Autodesk Inventor part; units mm, degrees
(part 2 of 2)
sketch "Sketch2" plane through (-209.3721, -28.8511, 0) normal (0, 0, -1) x (-1, 0, 0)
  line L0 (-33.637, 21.3645) -> (-33.637, 17.6082) projected
  line L1 (-48.637, 21.3645) -> (-33.637, 21.3645) projected
  line L2 (-48.637, 17.6082) -> (-48.637, 21.3645) projected
  line L3 (-48.637, 17.6082) -> (-33.637, 17.6082) projected
  line L4 (-49.637, 20.8382) -> (-49.637, 18.1345) projected
  line L5 (-32.637, 18.1345) -> (-32.637, 20.8382) projected
  line L6 (-26.637, 21.1086) -> (-26.637, 17.8642) projected
  line L7 (-25.437, 17.2326) -> (-25.437, 21.7402) projected
  line L8 (-4.837, 21.7402) -> (-4.837, 17.2326) projected
  line L9 (-25.437, 21.7402) -> (-4.837, 21.7402) projected
  line L10 (-25.437, 17.2326) -> (-25.437, 21.7402) projected
  line L11 (-25.437, 17.2326) -> (-4.837, 17.2326) projected
  line L12 (-3.637, 17.8642) -> (-3.637, 21.1086) projected
  line L13 (2.363, 17.6864) -> (2.363, 21.2864) projected
  spline S0 degree 2 poles (3.563, 17.2326) (3.5291, 17.2777) (2.2161, 19.0571) (2.9463, 20.9193) (3.563, 21.7402) knots 3.326026 3.326026 3.326026 3.405258 7.652604 9.28848 9.28848 9.28848 weights 9.554217 9.619621 13.096193 10.904595 9.554217 projected
  line L14 (3.563, 17.2326) -> (46.163, 17.2326) projected
  line L15 (46.163, 21.7402) -> (46.163, 17.2326) projected
  line L16 (3.563, 21.7402) -> (46.163, 21.7402) projected
  line L17 (47.363, 21.2864) -> (47.363, 17.6864) projected
  circle A0 centre (29.9929, 5.3328) radius 3.7 projected
  circle A1 centre (29.9929, 5.3328) radius 5.3 projected
  circle A2 centre (29.9929, 5.3328) radius 5.8 projected
  circle A3 centre (45.4783, 5.604) radius 5.8 projected
  circle A4 centre (45.4783, 5.604) radius 5.3 projected
  line L18 (2.363, 14.1086) -> (2.363, 10.8642) projected
  line L19 (18.363, 10.8642) -> (18.363, 14.1086) projected
  line L20 (18.363, 3.8642) -> (18.363, 7.1086) projected
  line L21 (2.363, 7.1086) -> (2.363, 3.8642) projected
  line L22 (-3.637, 10.8642) -> (-3.637, 14.1086) projected
  line L23 (-26.637, 14.1086) -> (-26.637, 10.8642) projected
  line L24 (-26.637, 7.1086) -> (-26.637, 3.8642) projected
  line L25 (-3.637, 3.8642) -> (-3.637, 7.1086) projected
  line L26 (-3.637, -3.1358) -> (-3.637, 0.1086) projected
  line L27 (-26.637, 0.1086) -> (-26.637, -3.1358) projected
  line L28 (-32.637, 0.1345) -> (-32.637, 2.8382) projected
  line L29 (-32.637, 6.1345) -> (-32.637, 8.8382) projected
  line L30 (-32.637, 12.1345) -> (-32.637, 14.8382) projected
  line L31 (-49.637, 14.8382) -> (-49.637, 12.1345) projected
  line L32 (-49.637, 8.8382) -> (-49.637, 6.1345) projected
  line L33 (-49.637, 2.8382) -> (-49.637, 0.1345) projected
  circle A5 centre (-40.7352, -15) radius 3.15 projected
  circle A6 centre (-26.7352, -15) radius 3.15 projected
  arc A7 (-40.7352, -11.1) -> (-40.7352, -18.9) centre (-40.7352, -15) ccw projected
  line L34 (-40.7352, -18.9) -> (-26.7352, -18.9) projected
  arc A8 (-26.7352, -18.9) -> (-26.7352, -11.1) centre (-26.7352, -15) ccw projected
  line L35 (-26.7352, -11.1) -> (-40.7352, -11.1) projected
  arc A9 (-40.7352, -10.5) -> (-40.7352, -19.5) centre (-40.7352, -15) ccw projected
  arc A10 (-26.7352, -19.5) -> (-26.7352, -10.5) centre (-26.7352, -15) ccw projected
  arc A11 (-3.0622, -10.5) -> (-3.0622, -19.5) centre (-3.0622, -15) ccw projected
  circle A12 centre (-3.0622, -15) radius 3.15 projected
  circle A13 centre (10.9378, -15) radius 3.15 projected
  arc A14 (-3.0622, -11.1) -> (-3.0622, -18.9) centre (-3.0622, -15) ccw projected
  line L36 (10.9378, -18.9) -> (-3.0622, -18.9) projected
  arc A15 (10.9378, -18.9) -> (10.9378, -11.1) centre (10.9378, -15) ccw projected
  line L37 (-3.0622, -11.1) -> (10.9378, -11.1) projected
  arc A16 (10.9378, -19.5) -> (10.9378, -10.5) centre (10.9378, -15) ccw projected
  line L38 (25.5408, -13.2) -> (26.1532, -13.8124) projected
  line L39 (25.5408, -13.2) -> (22.9656, -13.2) projected
  line L40 (22.3532, -13.8124) -> (22.9656, -13.2) projected
  line L41 (22.3532, -13.8124) -> (22.3532, -16.3876) projected
  line L42 (22.9656, -17) -> (22.3532, -16.3876) projected
  line L43 (22.9656, -17) -> (25.5408, -17) projected
  line L44 (26.1532, -16.3876) -> (25.5408, -17) projected
  line L45 (26.1532, -16.3876) -> (26.1532, -13.8124) projected
  line L46 (33.3532, -16.3876) -> (32.7408, -17) projected
  line L47 (33.3532, -16.3876) -> (33.3532, -13.8124) projected
  line L48 (32.7408, -13.2) -> (33.3532, -13.8124) projected
  line L49 (32.7408, -13.2) -> (30.1656, -13.2) projected
  line L50 (29.5532, -13.8124) -> (30.1656, -13.2) projected
  line L51 (29.5532, -13.8124) -> (29.5532, -16.3876) projected
  line L52 (30.1656, -17) -> (29.5532, -16.3876) projected
  line L53 (30.1656, -17) -> (32.7408, -17) projected
  line L54 (-50, -27.5) -> (50, -27.5) projected
  arc A17 (50, -27.5) -> (60, -17.5) centre (50, -17.5) ccw projected
  line L55 (60, -17.5) -> (60, 17.5) projected
  arc A18 (60, 17.5) -> (50, 27.5) centre (50, 17.5) ccw projected
  line L56 (50, 27.5) -> (-50, 27.5) projected
  arc A19 (-50, 27.5) -> (-60, 17.5) centre (-50, 17.5) ccw projected
  line L57 (-60, 17.5) -> (-60, -17.5) projected
  arc A20 (-60, -17.5) -> (-50, -27.5) centre (-50, -17.5) ccw projected
  line L58 (-60, 19.9645) -> (-60, 18.9645)
  line L59 (60, 18.9645) -> (60, 19.9645)
  line L60 (-60, 5.0086) -> (-60, 6.0086)
  line L61 (60, 6.0086) -> (60, 5.0086)
  line L62 (51.2642, 6.0086) -> (60, 6.0086)
  line L63 (60, 5.0086) -> (51.2477, 5.0086)
  line L64 (35.7534, 6.0086) -> (39.6925, 6.0086)
  line L65 (39.709, 5.0086) -> (35.7838, 5.0086)
  line L66 (24.2019, 5.0086) -> (18.363, 5.0086)
  line L67 (18.363, 6.0086) -> (24.2324, 6.0086)
  line L68 (-30.137, 19.9645) -> (-29.137, 19.9645)
  line L69 (-29.137, 19.9645) -> (-29.137, -2.0358)
  line L70 (-29.137, -2.0358) -> (-30.137, -2.0358)
  line L71 (-30.137, -2.0358) -> (-30.137, 19.9645)
  line L72 (18.363, 12.0086) -> (60, 12.0086)
  line L73 (60, 12.0086) -> (60, 13.0086)
  line L74 (60, 13.0086) -> (18.363, 13.0086)
  line L75 (18.363, 13.0086) -> (18.363, 12.0086)
  line L76 (-29.137, 12.0086) -> (-29.137, 13.0086)
  line L77 (18.363, 13.0086) -> (18.363, 12.0086)
  line L78 (-3.637, 4.9642) -> (2.5322, 4.9642)
  line L79 (2.5322, 4.9642) -> (2.5322, 5.9642)
  line L80 (2.5322, 5.9642) -> (-3.637, 5.9642)
  line L81 (-3.637, 5.9642) -> (-3.637, 4.9642)
  line L82 (-26.637, 4.9642) -> (-30.137, 4.9642)
  line L83 (-30.137, 4.9642) -> (-30.137, 5.9642)
  line L84 (-30.137, 5.9642) -> (-26.637, 5.9642)
  line L85 (-26.637, 5.9642) -> (-26.637, 4.9642)
  line L86 (-26.637, -1.0358) -> (-29.137, -1.0358)
  line L87 (-29.137, -1.0358) -> (-29.137, -2.0358)
  line L88 (-29.137, -2.0358) -> (-26.637, -2.0358)
  line L89 (-26.637, -2.0358) -> (-26.637, -1.0358)
  line L90 (-32.637, 1.9882) -> (-29.137, 1.9882)
  line L91 (-29.137, 1.9882) -> (-29.137, 0.9882)
  line L92 (-29.137, 0.9882) -> (-32.637, 0.9882)
  line L93 (-32.637, 0.9882) -> (-32.637, 1.9882)
  line L94 (-32.637, 7.9882) -> (-29.137, 7.9882)
  line L95 (-29.137, 7.9882) -> (-29.137, 6.9882)
  line L96 (-29.137, 6.9882) -> (-32.637, 6.9882)
  line L97 (-32.637, 6.9882) -> (-32.637, 7.9882)
  line L98 (-32.637, 13.9882) -> (-30.137, 13.9882)
  line L99 (-30.137, 13.9882) -> (-30.137, 12.9882)
  line L100 (-30.137, 12.9882) -> (-32.637, 12.9882)
  line L101 (-32.637, 12.9882) -> (-32.637, 13.9882)
  line L102 (-49.637, 13.9882) -> (-60, 13.9882)
  line L103 (-60, 13.9882) -> (-60, 12.9882)
  line L104 (-60, 12.9882) -> (-49.637, 12.9882)
  line L105 (-32.637, 12.9882) -> (-32.637, 13.9882)
  line L106 (-49.637, 7.9882) -> (-60, 7.9882)
  line L107 (-60, 7.9882) -> (-60, 6.9882)
  line L108 (-60, 6.9882) -> (-49.637, 6.9882)
  line L109 (-32.637, 6.9882) -> (-32.637, 7.9882)
  line L110 (-49.637, 1.9882) -> (-60, 1.9882)
  line L111 (-60, 1.9882) -> (-60, 0.9882)
  line L112 (-60, 0.9882) -> (-49.637, 0.9882)
  line L113 (-0.437, 27.5) -> (-1.637, 27.5)
  line L114 (-1.637, 27.5) -> (-1.637, -2.0358)
  line L115 (-1.637, -2.0358) -> (-0.437, -2.0358)
  line L116 (-0.437, -2.0358) -> (-0.437, 27.5)
  line L117 (-3.637, -1.0358) -> (-1.637, -1.0358)
  line L118 (-1.637, -1.0358) -> (-1.637, -2.0358)
  line L119 (-1.637, -2.0358) -> (-3.637, -2.0358)
  line L120 (-3.637, -2.0358) -> (-3.637, -1.0358)
  line L121 (47.363, 18.9645) -> (60, 18.9645)
  line L122 (60, 19.9645) -> (47.363, 19.9645)
  line L123 (-29.137, 13.0086) -> (-26.637, 13.0086)
  line L124 (-3.637, 13.0086) -> (2.363, 13.0086)
  line L125 (2.363, 12.0086) -> (-3.637, 12.0086)
  line L126 (-26.637, 12.0086) -> (-29.137, 12.0086)
  line L127 (2.363, 19.9645) -> (-4.837, 19.9645)
  line L128 (-4.837, 18.9645) -> (2.363, 18.9645)
  line L129 (-25.437, 19.9645) -> (-32.637, 19.9645)
  line L130 (-49.637, 19.9645) -> (-60, 19.9645)
  line L131 (-60, 18.9645) -> (-49.637, 18.9645)
  line L132 (-32.637, 18.9645) -> (-25.437, 18.9645)
  line L133 (60, -15.5) -> (60, -14.5)
  line L134 (-60, -14.5) -> (-60, -15.5)
  line L135 (-14.2622, -14.5) -> (-13.0622, -14.5)
  line L136 (-13.0622, -14.5) -> (-13.0622, -27.5)
  line L137 (-13.0622, -27.5) -> (-14.2622, -27.5)
  line L138 (-14.2622, -27.5) -> (-14.2622, -14.5)
  line L139 (18.1532, -14.5) -> (19.3532, -14.5)
  line L140 (19.3532, -14.5) -> (19.3532, -27.5)
  line L141 (19.3532, -27.5) -> (18.1532, -27.5)
  line L142 (18.1532, -27.5) -> (18.1532, -14.5)
  line L143 (50.8547, -15.5) -> (60, -15.5)
  line L144 (39.8194, -14.5) -> (33.3532, -14.5)
  line L145 (33.3532, -15.5) -> (39.8336, -15.5)
  line L146 (29.5532, -14.5) -> (26.1532, -14.5)
  line L147 (26.1532, -15.5) -> (29.5532, -15.5)
  line L148 (22.3532, -14.5) -> (15.41, -14.5)
  line L149 (15.41, -15.5) -> (22.3532, -15.5)
  line L150 (-60, -15.5) -> (-45.2073, -15.5)
  line L151 (-7.5343, -14.5) -> (-22.2631, -14.5)
  line L152 (-45.2073, -14.5) -> (-60, -14.5)
  line L153 (-22.2631, -15.5) -> (-7.5343, -15.5)
  circle A21 centre (45.2028, -14.9239) radius 5.4 projected
  line L154 (60, -15.5) -> (50.5719, -15.5)
  line L155 (50.5861, -14.5) -> (60, -14.5)
  line L156 (60, -14.5) -> (60, -15.5)
  point P0 (-209.3721, 28.8511)
  point P1 (-30.887, 6.9882)
  point P2 (-14.2622, -21)
  point P3 (18.1532, -15.5)
  point P4 (18.1532, -27.5)
  point P5 (19.3532, -15.5)
  point P6 (19.3532, -14.5)
  point P7 (-14.2622, -15.5)
  point P8 (-14.2622, -27.5)
  point P9 (-13.0622, -15.5)
  point P10 (-13.0622, -14.5)
  point P11 (-60, -14.5)
  point P12 (-60, -15.5)
  point P13 (-60, 1.9882)
  point P14 (-60, 7.9882)
  point P15 (-60, 13.9882)
  point P16 (-59.8922, 18.9645)
  point P17 (-59.6915, 19.9645)
  point P18 (-29.137, -2.0358)
  point P19 (-26.637, -2.0358)
  point P20 (-29.137, -1.0358)
  point P21 (-29.137, 4.9642)
  point P22 (-26.637, 5.9642)
  point P23 (-29.137, 5.9642)
  point P24 (-29.137, 12.0086)
  point P25 (-29.137, 18.9645)
  point P26 (-26.637, 18.9645)
  point P27 (-26.637, 19.9645)
  point P28 (-29.137, 19.9645)
  point P29 (-30.137, 18.9645)
  point P30 (-30.137, 13.9882)
  point P31 (-32.637, 12.9882)
  point P32 (-30.137, 7.9882)
  point P33 (-32.637, 6.9882)
  point P34 (-30.137, 6.9882)
  point P35 (-30.137, 1.9882)
  point P36 (-32.637, 0.9882)
  point P37 (-30.137, 0.9882)
  point P38 (-0.437, 5.9642)
  point P39 (-0.437, 12.0086)
  point P40 (-0.437, 13.0086)
  point P41 (-0.437, 18.9645)
  point P42 (-0.437, 19.9645)
  point P43 (-1.637, 27.5)
  point P44 (-1.637, 19.9645)
  point P45 (-3.637, 19.9645)
  point P46 (-3.637, 18.9645)
  point P47 (-1.637, 18.9645)
  point P48 (-1.637, 13.0086)
  point P49 (-1.637, 12.0086)
  point P50 (-1.637, 5.9642)
  point P51 (-3.637, 5.9642)
  point P52 (-1.637, 4.9642)
  point P53 (-1.637, -1.0358)
  point P54 (-3.637, -2.0358)
  point P55 (-1.637, -2.0358)
  point P56 (-0.437, 4.9642)
  point P57 (59.6915, 19.9645)
  point P58 (59.8922, 18.9645)
  point P59 (18.363, 13.0086)
  point P60 (60, 12.0086)
  point P61 (60, 5.0086)
  point P62 (60, 6.0086)
  point P63 (60, -14.5)
  point P64 (50.8547, -15.5)
  point P65 (60, -15.5)
  point P66 (2.363, 4.9642)
  point P67 (2.363, 5.9642)
  dimension "d79" = 1
  dimension "d80" = 2.5
  dimension "d81" = 2.5
  dimension "d82" = 1
  dimension "d83" = 1.1
  dimension "d84" = 1.1444
  dimension "d85" = 1
  dimension "d86" = 1.1
  dimension "d87" = 1
  dimension "d89" = 1.2
  dimension "d90" = 2
  dimension "d91" = 1
  dimension "d92" = 0.85
  dimension "d93" = 0.8537
  dimension "d94" = 1
  dimension "d95" = 0.85
  dimension "d96" = 1
  dimension "d97" = 0.85
  dimension "d98" = 1
  dimension "d99" = 1.1
  dimension "d100" = 1.1444
  dimension "d101" = 1.1
  dimension "d102" = 1
  dimension "d103" = 1.1
  dimension "d104" = 1.1444
  dimension "d105" = 1.1444
  dimension "d106" = 1
  dimension "d107" = 0.8737
  dimension "d111" = 1.2
  dimension "d112" = 1.2
  dimension "d113" = 3
  dimension "d114" = 10
  dimension "d115" = 1
  dimension "d116" = 3.4
  dimension "d117" = 3.4
  dimension "d118" = 1
  constraints: 198 end point, 93 parallel, 62 point on line, 31 horizontal, 30 perpendicular, 27 horizontal alignment, 20 point on circle, 6 vertical alignment, 3 coincident, 2 midpoint
  measures "d79" distance between parallel lines of L69 L71
  measures "d80" distance between parallel lines of L5 L71
  measures "d81" distance between parallel lines of L69 L6
  measures "d82" distance between parallel lines of L72 L74
  measures "d83" distance from line of L19.end L74
  measures "d84" distance from line of L72 L19.start
  measures "d85" distance between parallel lines of L119 L117
  measures "d86" distance from line of L119 L26.start
  measures "d87" distance between parallel lines of L78 L80
  measures "d89" distance between parallel lines of L116 L114
  measures "d90" distance between parallel lines of L12 L114
  measures "d91" distance between parallel lines of L100 L98
  measures "d92" distance from line of L30.end L98
  measures "d93" distance from line of L100 L30.start
  measures "d94" distance from line of point (-30.887, 6.988) L94
  measures "d95" distance from line of L29.end L94
  measures "d96" distance between parallel lines of L92 L90
  measures "d97" distance of L28.end L90.start
  measures "d98" distance between parallel lines of L86 L88
  measures "d99" distance from line of L27.end L88
  measures "d100" distance of L27.start L86.start
  measures "d101" distance from line of L82 L24.end
  measures "d102" distance between parallel lines of L66 L67
  measures "d103" distance of L20.end L67.start
  measures "d104" distance from line of L20.start L66
  measures "d105" distance from line of L21.start L80
  measures "d106" distance between parallel lines of L131 L130
  measures "d107" distance from line of L4.start L130
  measures "d111" distance from line of L136 point (-14.262, -21)
  measures "d112" distance between parallel lines of L140 L142
  measures "d113" distance between parallel lines of L41 L140
  measures "d114" distance from line of A14.centre L136
  measures "d115" distance between parallel lines of L150 L152
  measures "d116" distance between parallel lines of L35 L152
  measures "d117" distance between parallel lines of L34 L150
  measures "d118" distance between parallel lines of L155 L143
extrude "Extrusion2" add sketch "Sketch2" against normal blind 1 contours L4 L131 A19 L130 | L56 L116 L127 L114 | L102 L31 L104 L57 | L127 L116 L128 L114 | L114 L128 L12 L127 | L127 L13 L128 L116 | L128 L116 L124 L114 | L106 L32 L108 L57 | A18 L121 L17 L122 | L124 L116 L125 L114 | L114 L125 L22 L124 | L124 L18 L125 L116 | L125 L116 L80 L114 | L114 L78 L25 L80 | L80 L116 L78 L114 | L55 L72 L19 L74 | L80 L21 L78 L116 | L78 L116 L115 L114 | L110 L33 L112 L57 | L114 L119 L26 L117 | L6 L132 L69 L129 | L55 L63 A3 L62 | L69 L132 L71 L68 | L152 A9 L150 L57 | L69 L94 L71 L132 | L71 L132 L5 L129 | L55 L143 L154 A21 L155 | A3 L65 A2 L64 | L123 L23 L126 L69 | L71 L100 L30 L98 | A21 L145 L47 L144 | A2 L66 L20 L67 | L69 L96 L71 L94 | L138 L153 L136 L54 | L69 L84 L71 L96 | L71 L96 L29 L94 | L153 A10 L151 L138 | L138 L135 L136 L153 | L54 L142 L149 L140 | L84 L24 L82 L69 | L69 L82 L71 L84 | L136 L151 A11 L153 | L149 L142 L139 L140 | L140 L148 L41 L149 | L69 L90 L71 L82 | L149 A16 L148 L142 | L69 L92 L71 L90 | L69 L70 L71 L92 | L71 L92 L28 L90 | L51 L147 L45 L146 | L86 L27 L88 L69
sketch "Sketch3" plane through (-357.3721, -11.3511, 0) normal (0, 1, 0) x (1, 0, 0)
  line L0 (28.7026, -1.5) -> (0, -1.5) projected
  line L1 (28.7026, -1.5) -> (26.7026, -1.5)
  line L2 (26.7026, -1.5) -> (26.7026, -3.5)
  line L3 (26.7026, -3.5) -> (28.7026, -3.5)
  line L4 (28.7026, -3.5) -> (28.7026, -1.5)
  line L5 (28.7026, -2.5) -> (28.1253, -1.5)
  line L6 (28.7026, -3.5) -> (26.7026, -1.5)
  line L7 (45.4684, -1.5) -> (1, -1.5)
  line L8 (45.4684, -1.5) -> (43.4684, -1.5)
  line L9 (43.4684, -1.5) -> (43.4684, -3.5)
  line L10 (43.4684, -3.5) -> (45.4684, -3.5)
  line L11 (45.4684, -3.5) -> (45.4684, -1.5)
  line L12 (45.4684, -2.5) -> (44.8911, -1.5)
  line L13 (45.4684, -3.5) -> (43.4684, -1.5)
  line L14 (62.2342, -1.5) -> (2, -1.5)
  line L15 (62.2342, -1.5) -> (60.2342, -1.5)
  line L16 (60.2342, -1.5) -> (60.2342, -3.5)
  line L17 (60.2342, -3.5) -> (62.2342, -3.5)
  line L18 (62.2342, -3.5) -> (62.2342, -1.5)
  line L19 (62.2342, -2.5) -> (61.6569, -1.5)
  line L20 (62.2342, -3.5) -> (60.2342, -1.5)
  line L21 (59.2342, -5.0609) -> (59.2342, 6.5086) construction
  line L22 (56.2342, 0) -> (56.2342, -1.5) projected
  line L23 (62.2342, 0) -> (62.2342, -1.5) projected
  line L24 (56.2342, -2.5) -> (56.8116, -1.5)
  line L25 (58.2342, -1.5) -> (58.2342, -3.5)
  line L26 (58.2342, -3.5) -> (56.2342, -3.5)
  line L27 (56.2342, -3.5) -> (56.2342, -1.5)
  line L28 (56.2342, -3.5) -> (58.2342, -1.5)
  line L29 (56.2342, -1.5) -> (116.4684, -1.5)
  line L30 (56.2342, -1.5) -> (58.2342, -1.5)
  line L31 (56.2342, 0) -> (56.2342, -1.5)
  line L32 (73, -3.5) -> (75, -1.5)
  line L33 (73, -2.5) -> (73.5774, -1.5)
  line L34 (73, -3.5) -> (73, -1.5)
  line L35 (73, -1.5) -> (75, -1.5)
  line L36 (75, -3.5) -> (73, -3.5)
  line L37 (75, -1.5) -> (75, -3.5)
  line L38 (39.4684, -3.5) -> (41.4684, -1.5)
  line L39 (39.4684, -2.5) -> (40.0458, -1.5)
  line L40 (39.4684, -3.5) -> (39.4684, -1.5)
  line L41 (39.4684, -1.5) -> (41.4684, -1.5)
  line L42 (41.4684, -3.5) -> (39.4684, -3.5)
  line L43 (41.4684, -1.5) -> (41.4684, -3.5)
  point P0 (357.3721, 0)
  point P1 (26.7026, -1.5)
  point P2 (41.4684, -1.5)
  point P3 (40.0458, -1.5)
  point P4 (43.4684, -1.5)
  point P5 (44.8911, -1.5)
  point P6 (58.2342, -1.5)
  point P7 (56.8116, -1.5)
  point P8 (61.6569, -1.5)
  point P9 (60.2342, -1.5)
  point P10 (75, -1.5)
  point P11 (73.5774, -1.5)
  dimension "d121" = 2
  dimension "d122" = 2
  dimension "d123" = 60
  dimension "d124" = 2
  dimension "d125" = 2
  dimension "d126" = 60
  dimension "d127" = 2
  dimension "d128" = 2
  dimension "d129" = 60
  dimension "d130" = 3
  dimension "d131" = 3
  dimension "d132" = 2
  dimension "d133" = 2
  dimension "d134" = 60
  dimension "d135" = 1
  dimension "d136" = 2
  dimension "d137" = 2
  dimension "d138" = 60
  dimension "d139" = 1
  constraints: 82 end point, 11 coincident, 9 symmetric about line, 6 parallel, 6 perpendicular, 6 point on line, 5 midpoint, 3 horizontal, 1 vertical
  measures "d121" distance between parallel lines of L2 L4
  measures "d122" distance between parallel lines of L0 L3
  measures "d123" angle of L0 L5
  measures "d124" distance between parallel lines of L9 L11
  measures "d125" distance between parallel lines of L7 L10
  measures "d126" angle of L7 L12
  measures "d127" distance between parallel lines of L16 L18
  measures "d128" distance between parallel lines of L14 L17
  measures "d129" angle of L14 L19
  measures "d130" distance between parallel lines of L21 L22
  measures "d131" distance between parallel lines of L23 L21
  measures "d132" distance between parallel lines of L35 L36
  measures "d133" distance between parallel lines of L34 L37
  measures "d134" angle of L33 L35
  measures "d135" distance of L32.start L33.start
  measures "d136" distance between parallel lines of L41 L42
  measures "d137" distance between parallel lines of L40 L43
  measures "d138" angle of L39 L41
  measures "d139" distance of L40.start L39.start
extrude "Extrusion3" add sketch "Sketch3" against normal up to surface (1.2 mm away) contours L14 L19 L18 L20 | L7 L12 L11 L13 | L5 L4 L6 L0 | L7 L38 L40 L39 | L14 L28 L27 L24 | L29 L32 L34 L33
sketch "Sketch4" plane through (-357.3721, -45.1511, 0) normal (0, 1, 0) x (1, 0, 0)
  line L0 (62.7103, -3.5) -> (64.7103, -1.5)
  line L1 (62.7103, -2.5) -> (63.2877, -1.5)
  line L2 (62.7103, -3.5) -> (62.7103, -1.5)
  line L3 (62.7103, -1.5) -> (64.7103, -1.5)
  line L4 (64.7103, -3.5) -> (62.7103, -3.5)
  line L5 (64.7103, -1.5) -> (64.7103, -3.5)
  line L6 (45.9075, -3.5) -> (45.9075, -1.5)
  line L7 (45.9075, -2.5) -> (46.4849, -1.5)
  line L8 (45.9075, -1.5) -> (47.9075, -1.5)
  line L9 (47.9075, -1.5) -> (47.9075, -3.5)
  line L10 (47.9075, -3.5) -> (45.9075, -3.5)
  line L11 (45.9075, -3.5) -> (47.9075, -1.5)
  line L12 (29.1787, -3.5) -> (29.1787, -1.5)
  line L13 (29.1787, -2.5) -> (29.7561, -1.5)
  line L14 (29.1787, -1.5) -> (31.1787, -1.5)
  line L15 (31.1787, -1.5) -> (31.1787, -3.5)
  line L16 (31.1787, -3.5) -> (29.1787, -3.5)
  line L17 (29.1787, -3.5) -> (31.1787, -1.5)
  line L18 (18.4129, -1.5) -> (16.4129, -1.5)
  line L19 (16.4129, -1.5) -> (16.4129, -3.5)
  line L20 (16.4129, -3.5) -> (18.4129, -3.5)
  line L21 (18.4129, -3.5) -> (18.4129, -1.5)
  line L22 (18.4129, -2.5) -> (17.8356, -1.5)
  line L23 (18.4129, -3.5) -> (16.4129, -1.5)
  line L24 (33.1787, -1.5) -> (33.1787, -3.5)
  line L25 (33.1787, -3.5) -> (35.1787, -3.5)
  line L26 (35.1787, -3.5) -> (33.1787, -1.5)
  line L27 (35.1787, -3.5) -> (35.1787, -1.5)
  line L28 (35.1787, -2.5) -> (34.6014, -1.5)
  line L29 (35.1787, -1.5) -> (33.1787, -1.5)
  line L30 (51.9445, -3.5) -> (51.9445, -1.5)
  line L31 (51.9445, -2.5) -> (51.3672, -1.5)
  line L32 (51.9445, -1.5) -> (49.9445, -1.5)
  line L33 (49.9445, -1.5) -> (49.9445, -3.5)
  line L34 (49.9445, -3.5) -> (51.9445, -3.5)
  line L35 (51.9445, -3.5) -> (49.9445, -1.5)
  point P0 (357.3721, 0)
  dimension "d142" = 2
  dimension "d143" = 2
  dimension "d144" = 60
  dimension "d145" = 1
  dimension "d146" = 2
  dimension "d147" = 2
  dimension "d148" = 60
  dimension "d149" = 1
  dimension "d150" = 2
  dimension "d151" = 2
  dimension "d152" = 60
  dimension "d153" = 1
  dimension "d154" = 2
  dimension "d155" = 2
  dimension "d156" = 60
  dimension "d157" = 2
  dimension "d158" = 2
  dimension "d159" = 60
  dimension "d160" = 2
  dimension "d161" = 2
  dimension "d162" = 60
  constraints: 72 end point, 17 coincident, 6 midpoint, 6 parallel, 6 perpendicular, 6 point on line, 3 horizontal
  measures "d142" distance between parallel lines of L3 L4
  measures "d143" distance between parallel lines of L2 L5
  measures "d144" angle of L1 L3
  measures "d145" distance of L2.start L1.start
  measures "d146" distance between parallel lines of L8 L10
  measures "d147" distance between parallel lines of L6 L9
  measures "d148" angle of L7 L8
  measures "d149" distance of L6.start L7.start
  measures "d150" distance between parallel lines of L14 L16
  measures "d151" distance between parallel lines of L12 L15
  measures "d152" angle of L13 L14
  measures "d153" distance of L12.start L13.start
  measures "d154" distance between parallel lines of L19 L21
  measures "d155" distance between parallel lines of L20 L18
  measures "d156" angle of L18 L22
  measures "d157" distance between parallel lines of L24 L27
  measures "d158" distance between parallel lines of L25 L29
  measures "d159" angle of L29 L28
  measures "d160" distance between parallel lines of L33 L30
  measures "d161" distance between parallel lines of L34 L32
  measures "d162" angle of L32 L31
extrude "Extrusion4" add sketch "Sketch4" against normal up to surface (1.2 mm away) contours L2 L1 L3 L0 | L6 L7 L8 L11 | L12 L13 L14 L17 | L22 L21 L23 L18 | L29 L28 L27 L26 | L35 L32 L31 L30
sketch "Sketch6" plane through (-209.3721, -28.8511, 1) normal (0, 0, 1) x (1, 0, 0)
  line L0 (60, -15.5) -> (60, -14.5) projected
  line L1 (60, -14.5) -> (45.2073, -14.5) projected
  arc A0 (45.2073, -15.5) -> (45.2073, -14.5) centre (40.7352, -15) ccw projected
  line L2 (45.2073, -15.5) -> (60, -15.5) projected
  line L3 (14.2622, -27.5) -> (14.2622, -15.5) projected
  line L4 (14.2622, -15.5) -> (22.2631, -15.5) projected
  arc A1 (22.2631, -14.5) -> (22.2631, -15.5) centre (26.7352, -15) ccw projected
  line L5 (22.2631, -14.5) -> (7.5343, -14.5) projected
  arc A2 (7.5343, -15.5) -> (7.5343, -14.5) centre (3.0622, -15) ccw projected
  line L6 (7.5343, -15.5) -> (13.0622, -15.5) projected
  line L7 (13.0622, -15.5) -> (13.0622, -27.5) projected
  line L8 (13.0622, -27.5) -> (14.2622, -27.5) projected
  line L9 (-19.3532, -27.5) -> (-18.1532, -27.5) projected
  line L10 (-18.1532, -27.5) -> (-18.1532, -15.5) projected
  line L11 (-18.1532, -15.5) -> (-15.41, -15.5) projected
  arc A3 (-15.41, -14.5) -> (-15.41, -15.5) centre (-10.9378, -15) ccw projected
  line L12 (-15.41, -14.5) -> (-22.3532, -14.5) projected
  line L13 (-22.3532, -14.5) -> (-22.3532, -15.5) projected
  line L14 (-22.3532, -15.5) -> (-19.3532, -15.5) projected
  line L15 (-19.3532, -15.5) -> (-19.3532, -27.5) projected
  line L16 (-29.5532, -14.5) -> (-29.5532, -15.5) projected
  line L17 (-29.5532, -15.5) -> (-26.1532, -15.5) projected
  line L18 (-26.1532, -15.5) -> (-26.1532, -14.5) projected
  line L19 (-26.1532, -14.5) -> (-29.5532, -14.5) projected
  line L20 (-33.3532, -14.5) -> (-39.8194, -14.5) projected
  line L21 (-33.3532, -14.5) -> (-39.8194, -14.5) projected
  arc A4 (-39.8336, -15.5) -> (-39.8194, -14.5) centre (-45.2028, -14.9239) ccw projected
  line L22 (-39.8336, -15.5) -> (-33.3532, -15.5) projected
  line L23 (-33.3532, -15.5) -> (-33.3532, -14.5) projected
  arc A5 (-50.5861, -14.5) -> (-50.5719, -15.5) centre (-45.2028, -14.9239) ccw projected
  line L24 (-50.5861, -14.5) -> (-60, -14.5) projected
  line L25 (-60, -14.5) -> (-60, -15.5) projected
  line L26 (-60, -15.5) -> (-50.5719, -15.5) projected
  line L27 (-60, 6.0086) -> (-60, 5.0086) projected
  line L28 (-60, 5.0086) -> (-51.2477, 5.0086) projected
  arc A6 (-51.2642, 6.0086) -> (-51.2477, 5.0086) centre (-45.4783, 5.604) ccw projected
  line L29 (-51.2642, 6.0086) -> (-60, 6.0086) projected
  arc A7 (-39.709, 5.0086) -> (-39.6925, 6.0086) centre (-45.4783, 5.604) ccw projected
  line L30 (-39.709, 5.0086) -> (-35.7838, 5.0086) projected
  arc A8 (-35.7534, 6.0086) -> (-35.7838, 5.0086) centre (-29.9929, 5.3328) ccw projected
  line L31 (-35.7534, 6.0086) -> (-39.6925, 6.0086) projected
  line L32 (-18.363, 5.0086) -> (-18.363, 6.0086) projected
  line L33 (-18.363, 6.0086) -> (-24.2324, 6.0086) projected
  arc A9 (-24.2019, 5.0086) -> (-24.2324, 6.0086) centre (-29.9929, 5.3328) ccw projected
  line L34 (-24.2019, 5.0086) -> (-18.363, 5.0086) projected
  line L35 (-18.363, 12.0086) -> (-18.363, 13.0086) projected
  line L36 (-18.363, 13.0086) -> (-60, 13.0086) projected
  line L37 (-60, 13.0086) -> (-60, 12.0086) projected
  line L38 (-60, 12.0086) -> (-18.363, 12.0086) projected
  line L39 (-47.363, 18.9645) -> (-47.363, 19.9645) projected
  line L40 (-47.363, 19.9645) -> (-59.6915, 19.9645) projected
  arc A10 (-59.6915, 19.9645) -> (-59.8922, 18.9645) centre (-50, 17.5) ccw projected
  line L41 (-59.8922, 18.9645) -> (-47.363, 18.9645) projected
  line L42 (0.437, 5.9642) -> (-2.363, 5.9642) projected
  line L43 (-2.363, 4.9642) -> (0.437, 4.9642) projected
  line L44 (0.437, 4.9642) -> (0.437, -2.0358) projected
  line L45 (0.437, -2.0358) -> (3.637, -2.0358) projected
  line L46 (3.637, -2.0358) -> (3.637, -1.0358) projected
  line L47 (3.637, -1.0358) -> (1.637, -1.0358) projected
  line L48 (1.637, -1.0358) -> (1.637, 4.9642) projected
  line L49 (1.637, 4.9642) -> (3.637, 4.9642) projected
  line L50 (3.637, 4.9642) -> (3.637, 5.9642) projected
  line L51 (3.637, 5.9642) -> (1.637, 5.9642) projected
  line L52 (1.637, 5.9642) -> (1.637, 12.0086) projected
  line L53 (1.637, 12.0086) -> (3.637, 12.0086) projected
  line L54 (3.637, 12.0086) -> (3.637, 13.0086) projected
  line L55 (3.637, 13.0086) -> (1.637, 13.0086) projected
  line L56 (1.637, 13.0086) -> (1.637, 18.9645) projected
  line L57 (1.637, 18.9645) -> (3.637, 18.9645) projected
  line L58 (3.637, 18.9645) -> (3.637, 19.9645) projected
  line L59 (3.637, 19.9645) -> (1.637, 19.9645) projected
  line L60 (1.637, 19.9645) -> (1.637, 27.5) projected
  line L61 (1.637, 27.5) -> (0.437, 27.5) projected
  line L62 (0.437, 27.5) -> (0.437, 19.9645) projected
  line L63 (0.437, 19.9645) -> (-2.363, 19.9645) projected
  line L64 (-2.363, 19.9645) -> (-2.363, 18.9645) projected
  line L65 (-2.363, 18.9645) -> (0.437, 18.9645) projected
  line L66 (0.437, 18.9645) -> (0.437, 13.0086) projected
  line L67 (0.437, 13.0086) -> (-2.363, 13.0086) projected
  line L68 (-2.363, 13.0086) -> (-2.363, 12.0086) projected
  line L69 (-2.363, 12.0086) -> (0.437, 12.0086) projected
  line L70 (0.437, 12.0086) -> (0.437, 5.9642) projected
  line L71 (26.637, -2.0358) -> (30.137, -2.0358) projected
  line L72 (30.137, -2.0358) -> (30.137, 0.9882) projected
  line L73 (30.137, 0.9882) -> (32.637, 0.9882) projected
  line L74 (32.637, 0.9882) -> (32.637, 1.9882) projected
  line L75 (32.637, 1.9882) -> (30.137, 1.9882) projected
  line L76 (30.137, 1.9882) -> (30.137, 6.9882) projected
  line L77 (30.137, 6.9882) -> (32.637, 6.9882) projected
  line L78 (32.637, 6.9882) -> (32.637, 7.9882) projected
  line L79 (32.637, 7.9882) -> (30.137, 7.9882) projected
  line L80 (30.137, 7.9882) -> (30.137, 12.9882) projected
  line L81 (30.137, 12.9882) -> (32.637, 12.9882) projected
  line L82 (32.637, 12.9882) -> (32.637, 13.9882) projected
  line L83 (32.637, 13.9882) -> (30.137, 13.9882) projected
  line L84 (30.137, 13.9882) -> (30.137, 18.9645) projected
  line L85 (30.137, 18.9645) -> (32.637, 18.9645) projected
  line L86 (32.637, 18.9645) -> (32.637, 19.9645) projected
  line L87 (32.637, 19.9645) -> (26.637, 19.9645) projected
  line L88 (26.637, 19.9645) -> (26.637, 18.9645) projected
  line L89 (26.637, 18.9645) -> (29.137, 18.9645) projected
  line L90 (29.137, 18.9645) -> (29.137, 13.0086) projected
  line L91 (29.137, 13.0086) -> (26.637, 13.0086) projected
  line L92 (26.637, 13.0086) -> (26.637, 12.0086) projected
  line L93 (26.637, 12.0086) -> (29.137, 12.0086) projected
  line L94 (29.137, 12.0086) -> (29.137, 5.9642) projected
  line L95 (29.137, 5.9642) -> (26.637, 5.9642) projected
  line L96 (26.637, 5.9642) -> (26.637, 4.9642) projected
  line L97 (26.637, 4.9642) -> (29.137, 4.9642) projected
  line L98 (29.137, 4.9642) -> (29.137, -1.0358) projected
  line L99 (29.137, -1.0358) -> (26.637, -1.0358) projected
  line L100 (26.637, -1.0358) -> (26.637, -2.0358) projected
  line L101 (49.637, 7.9882) -> (49.637, 6.9882) projected
  line L102 (49.637, 6.9882) -> (60, 6.9882) projected
  line L103 (60, 6.9882) -> (60, 7.9882) projected
  line L104 (60, 7.9882) -> (49.637, 7.9882) projected
  line L105 (49.637, 1.9882) -> (49.637, 0.9882) projected
  line L106 (49.637, 0.9882) -> (60, 0.9882) projected
  line L107 (60, 0.9882) -> (60, 1.9882) projected
  line L108 (60, 1.9882) -> (49.637, 1.9882) projected
  line L109 (49.637, 13.9882) -> (49.637, 12.9882) projected
  line L110 (49.637, 12.9882) -> (60, 12.9882) projected
  line L111 (60, 12.9882) -> (60, 13.9882) projected
  line L112 (60, 13.9882) -> (49.637, 13.9882) projected
  line L113 (59.6915, 19.9645) -> (49.637, 19.9645) projected
  line L114 (49.637, 18.9645) -> (59.8922, 18.9645) projected
  line L115 (49.637, 19.9645) -> (49.637, 18.9645) projected
  line L116 (49.637, 18.9645) -> (59.8922, 18.9645) projected
  arc A11 (59.8922, 18.9645) -> (59.6915, 19.9645) centre (50, 17.5) ccw projected
  line L117 (59.6915, 19.9645) -> (49.637, 19.9645) projected
  line L118 (-2.363, 5.9642) -> (-2.363, 4.9642) projected
  point P0 (209.3721, 28.8511)
  point P1 (-39.8194, -14.5)
  point P2 (49.637, 19.9645)
  point P3 (49.637, 18.9645)
  point P4 (59.8922, 18.9645)
  point P5 (59.6915, 19.9645)
extrude "Extrusion6" add sketch "Sketch6" along normal blind 0.5 contours L2 A0 L1 L0 | L8 L7 L6 A2 L5 A1 L4 L3 | L15 L14 L13 L12 A3 L11 L10 L9 | L23 L22 A4 L20 | A5 L26 L25 L24 | L29 A6 L28 L27 | A7 L31 A8 L30 | L34 A9 L33 L32 | L38 L37 L36 L35 | L41 A10 L40 L39 | L70 L69 L68 L67 L66 L65 L64 L63 L62 L61 L60 L59 L58 L57 L56 L55 L54 L53 L52 L51 L50 L49 L48 L47 L46 L45 L44 L43 L118 L42 | L100 L99 L98 L97 L96 L95 L94 L93 L92 L91 L90 L89 L88 L87 L86 L85 L84 L83 L82 L81 L80 L79 L78 L77 L76 L75 L74 L73 L72 L71 | L104 L103 L102 L101 | L108 L107 L106 L105 | L112 L111 L110 L109 | A11 L114 L115 L113
sketch "Sketch7" plane through (0, 0, 1.5) normal (0, 0, 1) x (1, 0, 0)
  line L0 (-162.0859, -71.27) -> (-162.0859, -66.3511) projected
  line L1 (-162.0859, -66.3511) -> (-163.2859, -66.3511) projected
  line L2 (-163.2859, -66.3511) -> (-163.2859, -71.27) projected
  line L3 (-163.2859, -71.27) -> (-162.0859, -71.27) projected
  line L4 (-133.3721, -74.8511) -> (-139.3721, -74.8511) projected
  line L5 (-133.3721, -89.1511) -> (-139.3721, -89.1511) projected
  line L6 (-133.3721, -90.3511) -> (-133.3721, -89.1511) projected
  line L7 (-133.3721, -89.1511) -> (-139.3721, -89.1511) projected
  line L8 (-139.3721, -89.1511) -> (-139.3721, -90.3511) projected
  line L9 (-139.3721, -90.3511) -> (-133.3721, -90.3511) projected
  line L10 (-133.3721, -76.0511) -> (-133.3721, -74.8511) projected
  line L11 (-133.3721, -74.8511) -> (-139.3721, -74.8511) projected
  line L12 (-139.3721, -74.8511) -> (-139.3721, -76.0511) projected
  line L13 (-139.3721, -76.0511) -> (-133.3721, -76.0511) projected
  line L14 (-162.0859, -92.3511) -> (-163.2859, -92.3511) projected
  line L15 (-163.2859, -92.3511) -> (-163.2859, -98.3511) projected
  line L16 (-163.2859, -98.3511) -> (-162.0859, -98.3511) projected
  line L17 (-162.0859, -98.3511) -> (-162.0859, -92.3511) projected
  line L18 (-133.3721, -103.7611) -> (-133.3721, -102.5611) projected
  line L19 (-133.3721, -102.5611) -> (-139.3721, -102.5611) projected
  line L20 (-139.3721, -102.5611) -> (-139.3721, -103.7611) projected
  line L21 (-139.3721, -103.7611) -> (-133.3721, -103.7611) projected
  line L22 (-133.3721, -120.7611) -> (-133.3721, -119.5611) projected
  line L23 (-133.3721, -119.5611) -> (-139.3721, -119.5611) projected
  line L24 (-139.3721, -119.5611) -> (-139.3721, -120.7611) projected
  line L25 (-139.3721, -120.7611) -> (-133.3721, -120.7611) projected
  line L26 (-162.0859, -108.3511) -> (-163.2859, -108.3511) projected
  line L27 (-163.2859, -108.3511) -> (-163.2859, -115.3511) projected
  line L28 (-163.2859, -115.3511) -> (-162.0859, -115.3511) projected
  line L29 (-162.0859, -115.3511) -> (-162.0859, -108.3511) projected
  line L30 (-162.0859, -125.3511) -> (-163.2859, -125.3511) projected
  line L31 (-163.2859, -125.3511) -> (-163.2859, -145.7637) projected
  line L32 (-163.2859, -145.7637) -> (-166.0395, -145.7637) projected
  line L33 (-166.0395, -145.7637) -> (-166.0395, -146.3637) projected
  line L34 (-166.0395, -146.3637) -> (-154.7094, -146.3637) projected
  line L35 (-154.7094, -146.3637) -> (-154.7094, -145.7637) projected
  line L36 (-154.7094, -145.7637) -> (-162.0859, -145.7637) projected
  line L37 (-162.0859, -145.7637) -> (-162.0859, -125.3511) projected
  line L38 (-162.0859, -145.7637) -> (-162.0859, -125.3511) projected
  line L39 (-162.0859, -128.1493) -> (-163.2859, -128.1493)
  line L40 (-163.2859, -125.3511) -> (-163.2859, -145.7637) projected
  arc A0 (-262.3827, -133.7016) -> (-263.5827, -133.7963) centre (-262.8746, -135.1187) ccw projected
  line L41 (-262.3827, -133.7016) -> (-262.3827, -125.3511) projected
  line L42 (-262.3827, -125.3511) -> (-263.5827, -125.3511) projected
  line L43 (-263.5827, -125.3511) -> (-263.5827, -133.7963) projected
  line L44 (-262.3827, -133.7016) -> (-262.3827, -125.3511) projected
  line L45 (-262.3827, -127.352) -> (-263.5827, -127.352)
  line L46 (-263.5827, -125.3511) -> (-263.5827, -133.7963) projected
  line L47 (-231.5215, -66.3511) -> (-232.7215, -66.3511) projected
  line L48 (-232.7215, -66.3511) -> (-232.7215, -76.2874) projected
  line L49 (-232.7215, -76.2874) -> (-231.5215, -76.2008) projected
  line L50 (-231.5215, -76.2008) -> (-231.5215, -66.3511) projected
  line L51 (-347.4137, -87.3511) -> (-348.6137, -87.3511) projected
  line L52 (-348.6137, -87.3511) -> (-348.6137, -88.7511) projected
  line L53 (-348.6137, -88.7511) -> (-357.3721, -88.7511) projected
  line L54 (-357.3721, -88.7511) -> (-357.3721, -89.9511) projected
  line L55 (-357.3721, -89.9511) -> (-348.6137, -89.9511) projected
  line L56 (-348.6137, -89.9511) -> (-348.6137, -91.3511) projected
  line L57 (-348.6137, -91.3511) -> (-347.4137, -91.3511) projected
  line L58 (-347.4137, -91.3511) -> (-347.4137, -89.9511) projected
  line L59 (-347.4137, -89.9511) -> (-307.5721, -89.9511) projected
  line L60 (-307.5721, -89.9511) -> (-307.5721, -106.9247) projected
  line L61 (-307.5721, -106.9247) -> (-306.3721, -106.9247) projected
  line L62 (-306.3721, -106.9247) -> (-306.3721, -89.9511) projected
  line L63 (-306.3721, -89.9511) -> (-281.5721, -89.9511) projected
  line L64 (-281.5721, -89.9511) -> (-281.5721, -106.9247) projected
  line L65 (-281.5721, -106.9247) -> (-280.3721, -106.9247) projected
  line L66 (-280.3721, -106.9247) -> (-280.3721, -89.9511) projected
  line L67 (-280.3721, -89.9511) -> (-232.7215, -89.9511) projected
  line L68 (-232.7215, -89.9511) -> (-232.7215, -98.3511) projected
  line L69 (-232.7215, -98.3511) -> (-231.5215, -98.3511) projected
  line L70 (-231.5215, -98.3511) -> (-231.5215, -87.5014) projected
  line L71 (-231.5215, -87.5014) -> (-232.7215, -87.4147) projected
  line L72 (-232.7215, -87.4147) -> (-232.7215, -88.7511) projected
  line L73 (-232.7215, -88.7511) -> (-313.8821, -88.7511) projected
  line L74 (-313.8821, -88.7511) -> (-313.8821, -87.3511) projected
  line L75 (-313.8821, -87.3511) -> (-315.0821, -87.3511) projected
  line L76 (-315.0821, -87.3511) -> (-315.0821, -88.7511) projected
  line L77 (-315.0821, -88.7511) -> (-330.6479, -88.7511) projected
  line L78 (-330.6479, -88.7511) -> (-330.6479, -87.3511) projected
  line L79 (-330.6479, -87.3511) -> (-331.8479, -87.3511) projected
  line L80 (-331.8479, -87.3511) -> (-331.8479, -88.7511) projected
  line L81 (-331.8479, -88.7511) -> (-347.4137, -88.7511) projected
  line L82 (-347.4137, -88.7511) -> (-347.4137, -87.3511) projected
  line L83 (-232.7215, -88.7511) -> (-313.8821, -88.7511) projected
  line L84 (-232.7215, -88.7511) -> (-232.7215, -89.9511)
  line L85 (-280.3721, -89.9511) -> (-232.7215, -89.9511) projected
  line L86 (-232.7215, -88.7511) -> (-313.8821, -88.7511) projected
  line L87 (-313.8821, -88.7511) -> (-313.8821, -89.9511)
  line L88 (-307.5721, -120.7511) -> (-307.5721, -119.5511) projected
  line L89 (-307.5721, -119.5511) -> (-333.7763, -119.5511) projected
  line L90 (-333.7763, -119.5511) -> (-333.2977, -120.7511) projected
  line L91 (-333.2977, -120.7511) -> (-307.5721, -120.7511) projected
  line L92 (-344.0635, -120.7511) -> (-344.5421, -119.5511) projected
  line L93 (-344.5421, -119.5511) -> (-357.3721, -119.5511) projected
  line L94 (-357.3721, -119.5511) -> (-357.3721, -120.7511) projected
  line L95 (-357.3721, -120.7511) -> (-344.0635, -120.7511) projected
  line L96 (-335.729, -141.6513) -> (-336.2075, -140.4513) projected
  line L97 (-336.2075, -140.4513) -> (-357.3721, -140.4513) projected
  line L98 (-357.3721, -140.4513) -> (-357.3721, -141.6513) projected
  line L99 (-357.3721, -141.6513) -> (-335.729, -141.6513) projected
  line L100 (-307.5721, -141.6513) -> (-307.5721, -140.4513) projected
  line L101 (-307.5721, -140.4513) -> (-325.4417, -140.4513) projected
  line L102 (-325.4417, -140.4513) -> (-324.9632, -141.6513) projected
  line L103 (-324.9632, -141.6513) -> (-307.5721, -141.6513) projected
  line L104 (-322.3695, -189.3511) -> (-321.7866, -189.3511) projected
  line L105 (-321.7866, -189.3511) -> (-321.7866, -186.3511) projected
  line L106 (-321.7866, -186.3511) -> (-322.3695, -186.3511) projected
  line L107 (-322.3695, -186.3511) -> (-322.3695, -189.3511) projected
  line L108 (-231.5215, -125.3511) -> (-232.7215, -125.3511) projected
  line L109 (-232.7215, -125.3511) -> (-232.7215, -144.4446) projected
  line L110 (-232.7215, -144.4446) -> (-231.5215, -145.1375) projected
  line L111 (-231.5215, -145.1375) -> (-231.5215, -125.3511) projected
  line L112 (-232.7215, -129.1998) -> (-231.5215, -129.1998)
  line L113 (-231.5215, -145.1375) -> (-231.5215, -125.3511) projected
  line L114 (-231.5215, -108.3511) -> (-232.7215, -108.3511) projected
  line L115 (-232.7215, -108.3511) -> (-232.7215, -115.3511) projected
  line L116 (-232.7215, -115.3511) -> (-231.5215, -115.3511) projected
  line L117 (-231.5215, -115.3511) -> (-231.5215, -108.3511) projected
  line L118 (-162.0859, -71.27) -> (-162.0859, -66.3511) projected
  line L119 (-162.0859, -67.6199) -> (-163.2859, -67.7065)
  line L120 (-231.5215, -76.2008) -> (-231.5215, -66.3511) projected
  line L121 (-231.5215, -72.7213) -> (-232.7215, -72.7213)
  line L122 (-232.7215, -66.3511) -> (-232.7215, -76.2874) projected
  point P0 (0, 0)
  constraints: 14 end point, 12 point on line, 3 perpendicular, 2 horizontal, 1 vertical
extrude "Extrusion7" add sketch "Sketch7" along normal blind 1 contours L3 L2 L119 L0 | L10 L13 L12 L4 | L6 L9 L8 L5 | L17 L16 L15 L14 | L21 L20 L19 L18 | L25 L24 L23 L22 | L29 L28 L27 L26 | L37 L39 L31 L30 | L45 L43 L42 L41 | L50 L49 L48 L121 | L82 L81 L80 L79 L78 L77 L76 L75 L74 L87 L59 L58 L57 L56 L55 L54 L53 L52 L51 | L72 L71 L70 L69 L68 L84 | L91 L90 L89 L88 | L95 L94 L93 L92 | L99 L98 L97 L96 | L103 L102 L101 L100 | L111 L112 L109 L108 | L117 L116 L115 L114
sketch "Sketch8" plane through (-217.0721, -210.3511, 0) normal (-1, 0, 0) x (0, 0, 1)
  line L0 (1.5, 4) -> (1.5, 0) projected
  line L1 (1.5, 4) -> (1.5, 2.1589)
  line L2 (4.4747, 4) -> (1.5, 2.1589)
  line L3 (5.5807, 4) -> (1.5, 0.4951)
  line L4 (1.5, 0) -> (1.5, 4) projected
  line L5 (3.5, 4) -> (6.5, 4) projected
  point P0 (0, 210.3511)
  point P1 (1.5, 0.4951)
  constraints: 6 end point, 3 point on line
extrude "Extrusion8" add sketch "Sketch8" against normal up to surface (1.2 mm away)
sketch "Sketch9" plane through (0, 0, 2.5) normal (0, 0, 1) x (1, 0, 0)
  line L0 (-136.3721, -120.8014) -> (-136.3721, -74.8511)
  line L1 (-133.3721, -74.8511) -> (-139.3721, -74.8511) projected
  line L2 (-133.3721, -119.5611) -> (-139.3721, -119.5611) projected
  line L3 (-139.3721, -119.5611) -> (-139.3721, -120.7611) projected
  line L4 (-139.3721, -120.7611) -> (-133.3721, -120.7611) projected
  line L5 (-133.3721, -120.7611) -> (-133.3721, -119.5611) projected
  line L6 (-133.3721, -102.5611) -> (-139.3721, -102.5611) projected
  line L7 (-139.3721, -102.5611) -> (-139.3721, -103.7611) projected
  line L8 (-139.3721, -103.7611) -> (-133.3721, -103.7611) projected
  line L9 (-133.3721, -103.7611) -> (-133.3721, -102.5611) projected
  line L10 (-133.3721, -89.1511) -> (-139.3721, -89.1511) projected
  line L11 (-139.3721, -89.1511) -> (-139.3721, -90.3511) projected
  line L12 (-139.3721, -90.3511) -> (-133.3721, -90.3511) projected
  line L13 (-133.3721, -90.3511) -> (-133.3721, -89.1511) projected
  line L14 (-133.3721, -74.8511) -> (-139.3721, -74.8511) projected
  line L15 (-139.3721, -74.8511) -> (-139.3721, -76.0511) projected
  line L16 (-139.3721, -76.0511) -> (-133.3721, -76.0511) projected
  line L17 (-133.3721, -76.0511) -> (-133.3721, -74.8511) projected
  point P0 (0, 0)
  point P1 (-136.3721, -76.0511)
  point P2 (-136.3721, -90.3511)
  point P3 (-136.3721, -89.1511)
  point P4 (-136.3721, -103.7611)
  point P5 (-136.3721, -102.5611)
  point P6 (-136.3721, -120.7611)
  point P7 (-136.3721, -119.5611)
  constraints: 2 end point, 1 midpoint
extrude "Extrusion9" add sketch "Sketch9" along normal blind 1 contours L4 L3 L2 L0 | L16 L15 L1 L0 | L12 L11 L10 L0 | L8 L7 L6 L0
sketch "Sketch10" plane through (0, 0, 3.5) normal (0, 0, 1) x (1, 0, 0)
  line L0 (-139.3721, -90.3511) -> (-133.3721, -90.3511) projected
  line L1 (-137.8461, -90.3511) -> (-137.8461, -74.8839)
  line L2 (-139.3721, -90.3511) -> (-136.3721, -90.3511) projected
  line L3 (-136.3721, -90.3511) -> (-136.3721, -89.1511) projected
  line L4 (-136.3721, -89.1511) -> (-139.3721, -89.1511) projected
  line L5 (-139.3721, -89.1511) -> (-139.3721, -90.3511) projected
  line L6 (-139.3721, -76.0511) -> (-136.3721, -76.0511) projected
  line L7 (-136.3721, -76.0511) -> (-136.3721, -74.8511) projected
  line L8 (-136.3721, -74.8511) -> (-139.3721, -74.8511) projected
  line L9 (-139.3721, -74.8511) -> (-139.3721, -76.0511) projected
  point P0 (0, 0)
  point P1 (-137.8461, -89.1511)
  constraints: 2 end point, 1 point on line, 1 vertical
extrude "Extrusion10" add sketch "Sketch10" along normal blind 1 contours L5 L4 L1 L0 | L6 L9 L8 L7
sketch "Sketch11" plane through (0, 0, 2.5) normal (0, 0, 1) x (1, 0, 0)
  line L0 (-347.4137, -89.9511) -> (-313.8821, -89.9511) projected
  line L1 (-313.8821, -89.9511) -> (-313.8821, -87.3511) projected
  line L2 (-313.8821, -87.3511) -> (-315.0821, -87.3511) projected
  line L3 (-315.0821, -87.3511) -> (-315.0821, -88.7511) projected
  line L4 (-315.0821, -88.7511) -> (-330.6479, -88.7511) projected
  line L5 (-330.6479, -88.7511) -> (-330.6479, -87.3511) projected
  line L6 (-330.6479, -87.3511) -> (-331.8479, -87.3511) projected
  line L7 (-331.8479, -87.3511) -> (-331.8479, -88.7511) projected
  line L8 (-331.8479, -88.7511) -> (-347.4137, -88.7511) projected
  line L9 (-347.4137, -88.7511) -> (-347.4137, -87.3511) projected
  line L10 (-347.4137, -87.3511) -> (-348.6137, -87.3511) projected
  line L11 (-348.6137, -87.3511) -> (-348.6137, -88.7511) projected
  line L12 (-348.6137, -88.7511) -> (-357.3721, -88.7511) projected
  line L13 (-357.3721, -88.7511) -> (-357.3721, -89.9511) projected
  line L14 (-357.3721, -89.9511) -> (-348.6137, -89.9511) projected
  line L15 (-348.6137, -89.9511) -> (-348.6137, -91.3511) projected
  line L16 (-348.6137, -91.3511) -> (-347.4137, -91.3511) projected
  line L17 (-347.4137, -91.3511) -> (-347.4137, -89.9511) projected
  point P0 (0, 0)
extrude "Extrusion11" add sketch "Sketch11" along normal blind 1
